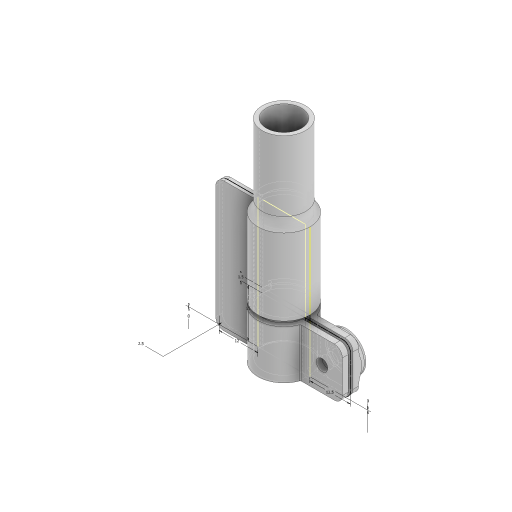
# Autodesk Inventor part: tube_clamp_r
Saved by Autodesk Inventor 2023 (Build 270158000, 158)
## iProperties
Created: 2023-02-09
Part Number: tube_clamp_r
Material: Generic
Document SubType Name: Modeling
Designer: Thomas
Density: 1 g/cm^3
Appearance: Default
Author: Thomas
Autodesk Inventor part; units mm, degrees
ref_plane "YZ Plane" through (0, 0, 0) normal (1, 0, 0) x (0, 1, 0)
ref_plane "XZ Plane" through (0, 0, 0) normal (0, 1, 0) x (-1, 0, 0)
ref_plane "XY Plane" through (0, 0, 0) normal (0, 0, 1) x (1, 0, 0)
sketch "Sketch1" plane through (0, 0, 0) normal (0, 1, 0) x (-1, 0, 0)
  circle A0 centre (0, 0) radius 6.55
  circle A1 centre (0, 0) radius 8
  dimension "d0" = 13.1
  dimension "d1" = 16
  dimension "d2" = 1.45
  constraints: 2 centre point, 2 coincident
  measures "d0" diameter of A0
  measures "d1" diameter of A1
  measures "d2" radial gap between concentric circles of A1 A0
extrude "Extrusion1" add sketch "Sketch1" along normal blind 40
sketch "Sketch2" plane through (0, 40, 0) normal (0, 1, 0) x (1, 0, 0)
  circle A0 centre (0, 0) radius 6.65
  circle A1 centre (0, 0) radius 5.4
  dimension "d5" = 13.3
  dimension "d6" = 10.8
  constraints: 2 centre point, 2 coincident
  measures "d5" diameter of A0
  measures "d6" diameter of A1
extrude "Extrusion2" add sketch "Sketch2" along normal blind 25
fillet "Fillet1" radius 5 1 edges at (-6.65, 40, 0)
fillet "Fillet2" radius 3 1 edges at (-5.4, 40, 0)
sketch "Sketch3" plane through (0, 0, 0) normal (0, 0, 1) x (1, 0, 0)
  line L0 (-8, 0) -> (-8, 40) projected
  line L1 (8, 0) -> (-8, 0) projected
  line L2 (8, 0) -> (8, 40) projected
  line L3 (-6.55, 40) -> (-6.55, 0) projected
  line L4 (6.55, 40) -> (6.55, 0) projected
  line L5 (-6.55, 40) -> (6.55, 40) projected
  line L6 (-6.55, 40) -> (-17.5, 40)
  line L7 (-20, 37.5) -> (-20, 2.5)
  line L8 (-20, 0) -> (-6.55, 0)
  line L9 (-6.55, 0) -> (-6.55, 40)
  line L10 (-6.55, 16.5) -> (8, 16.5)
  line L11 (8, 16.5) -> (8, 15)
  line L12 (8, 15) -> (-6.55, 15)
  line L13 (-6.55, 15) -> (-6.55, 16.5)
  line L14 (6.55, 15) -> (18, 15)
  line L15 (20.5, 12.5) -> (20.5, 2.5)
  line L16 (18, 0) -> (-17.5, 0)
  line L17 (6.55, 0) -> (6.55, 15)
  arc A0 (-20, 2.5) -> (-17.5, 0) centre (-17.5, 2.5) ccw
  arc A1 (-17.5, 40) -> (-20, 37.5) centre (-17.5, 37.5) ccw
  arc A2 (18, 0) -> (20.5, 2.5) centre (18, 2.5) ccw
  arc A3 (20.5, 12.5) -> (18, 15) centre (18, 12.5) ccw
  point P0 (0, 0)
  point P1 (-6.55, 15)
  dimension "d11" = 12
  dimension "d12" = 0
  dimension "d13" = 15
  dimension "d14" = 1.5
  dimension "d15" = 0
  dimension "d16" = 12.5
  dimension "d17" = 2.5
  constraints: 24 end point, 8 point on circle, 8 tangent, 6 parallel, 6 point on line, 4 centre point, 3 equal radius, 3 horizontal, 3 perpendicular
  measures "d11" distance between parallel lines of L7 L0
  measures "d12" distance between parallel lines of L1 L8
  measures "d13" distance between parallel lines of L1 L12
  measures "d14" distance between parallel lines of L10 L12
  measures "d15" distance between parallel lines of L16 L1
  measures "d16" distance between parallel lines of L2 L15
  measures "d17" radius of A0
extrude "Extrusion3" add sketch "Sketch3" along normal mid plane 2 contours L8 A0 L7 A1 L6 L0 | L0 L6 L3 L1
extrude "Extrusion4" add sketch "Sketch3" along normal mid plane 5 contours L4 L12 L2 L1 | L2 L14 A3 L15 A2 L16
sketch "Sketch4" plane through (0, 0, 0) normal (0, -1, 0) x (1, 0, 0)
  circle A0 centre (0, 0) radius 5.4 projected
  line L0 (20.5, -2.5) -> (20.5, 2.5) projected
  line L1 (20.5, 0.75) -> (0, 0.75)
  line L2 (0, 0.75) -> (0, -0.75)
  line L3 (0, -0.75) -> (20.5, -0.75)
  line L4 (20.5, -0.75) -> (20.5, 0.75)
  dimension "d22" = 1.5
  dimension "d23" = 0.75
  constraints: 8 end point, 2 parallel, 1 horizontal, 1 perpendicular, 1 point on line
  measures "d22" distance of L1.end L2.end
  measures "d23" distance from line of point (0, 0) L1
extrude "Extrusion5" cut sketch "Sketch4" against normal blind 15 contours A0 L3 L2 L1 | A0 L1 L0 L3 picked at (1.8, 0)
extrude "Extrusion6" cut sketch "Sketch3" along normal through all both and the other way through all contours L3 L10 L4 L12 | L4 L10 L2 L12
fillet "Fillet3" radius 0.5 2 edges at (-6.55, 15.75, 4.5932) (-6.55, 15.75, -4.5932)
fillet "Fillet4" radius 0.5 4 edges at (7.5993, 7.5, 2.5) (7.5993, 7.5, -2.5) (-7.9373, 20, -1) (-7.9373, 20, 1)
sketch "Sketch5" plane through (0, 0, -2.5) normal (0, 0, -1) x (-1, 0, 0)
  circle A0 centre (-14.25, 7.5) radius 6
  line L0 (-20.5, 12.5) -> (-20.5, 2.5) projected
  line L1 (-7.953, 15) -> (-18, 15) projected
  line L2 (-18, 0) -> (-7.953, 0) projected
  line L3 (-12.6046, 10.35) -> (-10.9591, 7.5)
  line L4 (-10.9591, 7.5) -> (-12.6046, 4.65)
  line L5 (-12.6046, 4.65) -> (-15.8954, 4.65)
  line L6 (-15.8954, 4.65) -> (-17.5409, 7.5)
  line L7 (-17.5409, 7.5) -> (-15.8954, 10.35)
  line L8 (-15.8954, 10.35) -> (-12.6046, 10.35)
  point P0 (0, 0)
  dimension "d30" = 12
  dimension "d31" = 6.25
  dimension "d32" = 15
  dimension "d33" = 7.5
  dimension "d34" = 5.7
  constraints: 12 end point, 1 centre point, 1 coincident, 1 parallel, 13 other
  measures "d30" diameter of A0
  measures "d31" distance from line of L0 A0.centre
  measures "d32" distance between parallel lines of L1 L2
  measures "d33" distance from line of A0.centre L2
  measures "d34" distance between parallel lines of L5 L8
extrude "Extrusion7" add sketch "Sketch5" along normal blind 2.5
fillet "Fillet5" radius 2 1 edges at (20.25, 7.5, -2.5)
sketch "Sketch6" plane through (0, 0, 2.5) normal (0, 0, 1) x (1, 0, 0)
  circle A0 centre (14.25, 7.5) radius 6 projected
  circle A1 centre (14.25, 7.5) radius 1.75
  point P0 (0, 0)
  dimension "d38" = 3.5
  constraints: 1 centre point, 1 coincident
  measures "d38" diameter of A1
extrude "Extrusion8" cut sketch "Sketch6" against normal through all contours A1
chamfer "Chamfer1" distance 1 angle 45 2 edges at (-0.3756, 0, 6.5392) (-0.3756, 0, -6.5392)
equation "\"d23\" = 0.5 * d22"
equation "\"d31\" = 0.5 * d16"
equation "\"d33\" = 0.5 * d32"
body "Solid1"
